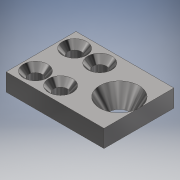
# Autodesk Inventor part: v2_bearing_insert_thick_round
Saved by Autodesk Inventor 2018 (Build 220112000, 112)
## iProperties
Created: 2017-04-27
Part Number: v2_bearing_insert_thick_round
Material: Stainless Steel, 440C
Document SubType Name: Modeling
Designer: richp
Density: 7.75 g/cm^3
Appearance: Semi-Polished
bearing_thickness: 0.125 in
Author: richp
Autodesk Inventor part; units mm, degrees
ref_plane "YZ Plane" through (0, 0, 0) normal (1, 0, 0) x (0, 1, 0)
sketch "Sketch1" plane through (0, 0, 0) normal (1, 0, 0) x (0, 1, 0)
  line L0 (-1.3067, 0) -> (7.8401, 0) construction
  line L1 (0, -10.9768) -> (0, 10.9768) construction
  line L2 (0, -1.7272) -> (0, -6.35)
  line L3 (0, -1.7272) -> (0, -1.7272)
  line L4 (0, -1.7272) -> (3.175, -3.5603)
  line L5 (3.175, -3.5603) -> (3.175, -6.35)
  line L6 (3.175, -6.35) -> (0, -6.35)
  circle A0 centre (3.3584, 0) radius 3.175 construction
  line L7 (2.5647, 7.8406) -> (4.1522, 7.8406) construction
  line L8 (4.1522, 7.8406) -> (4.1522, -7.8406) construction
  line L9 (4.1522, -7.8406) -> (2.5647, -7.8406) construction
  line L10 (2.5647, -7.8406) -> (2.5647, 7.8406) construction
  line L11 (2.5647, 7.8406) -> (4.1522, -7.8406) construction
  line L12 (4.1522, 7.8406) -> (2.5647, -7.8406) construction
  line L13 (0, 1.7272) -> (0, 6.35)
  line L14 (0, 1.7272) -> (0, 1.7272)
  line L15 (0, 1.7272) -> (3.175, 3.5603)
  line L16 (3.175, 3.5603) -> (3.175, 6.35)
  line L17 (3.175, 6.35) -> (0, 6.35)
  point P0 (0, 0)
  point P1 (2.3851, -3.0222)
  point P2 (2.3851, 3.0222)
  dimension "d12" = 60
  dimension "d13" = 0
  dimension "bearing_thickness" = 3.175
  dimension "d15" = 1.7272
  dimension "d17" = 6.35
  dimension "d18" = 1.5875
  dimension "d23" = 12.7
  dimension "d52" = 3.3584
  constraints: 32 end point, 5 symmetric about line, 4 perpendicular, 2 horizontal, 2 midpoint, 2 parallel, 2 point on circle, 2 point on line, 1 centre point, 1 coincident, 1 tangent
  measures "d12" angle of L1 L4
  measures "d13" distance of L2.start L3.end
  measures "bearing_thickness" distance of L5.end L2.end
  measures "d15" distance from line of point (0, 0) L3
  measures "d17" diameter of A0
  measures "d18" distance between parallel lines of L10 L8
  measures "d23" distance between parallel lines of L6 L17
  measures "d52" distance from line of L2 A0.centre
sketch "Sketch11" plane through (0, 0, 0) normal (1, 0, 0) x (0, 1, 0)
  line L0 (3.175, 6.35) -> (0, 6.35) projected
  line L1 (3.175, -6.35) -> (0, -6.35) projected
  line L2 (-1.3067, 0) -> (7.8401, 0) construction
  line L3 (0, -10.9768) -> (0, 10.9768) construction
  line L4 (3.175, 6.35) -> (3.175, 0.762)
  line L5 (3.175, 0.762) -> (0, 0.762)
  line L6 (0, 6.35) -> (0, 0.762)
  line L7 (3.175, -6.35) -> (0, -6.35)
  line L8 (0, 10.9768) -> (0, -10.9768) construction
  line L9 (3.175, -6.35) -> (3.175, -0.762)
  line L10 (3.175, -0.762) -> (0, -0.762)
  line L11 (0, -6.35) -> (0, -0.762)
  point P0 (0, 0)
  dimension "d54" = 5.588
  constraints: 16 end point, 4 symmetric about line, 2 perpendicular, 2 point on line, 1 vertical
  measures "d54" distance of L0.start L4.end
extrude "Extrusion4" add sketch "Sketch11" along normal blind 3.556 and the other way blind 14.224
sketch "Sketch17" plane through (3.556, 0, 0) normal (1, 0, 0) x (0, 0, -1)
  line L0 (-6.35, 3.175) -> (-0.762, 3.175) projected
  line L1 (-0.762, 3.175) -> (0.762, 3.175)
  line L2 (0.762, 3.175) -> (0.762, 0)
  line L3 (0.762, 0) -> (-0.762, 0)
  line L4 (-0.762, 0) -> (-0.762, 3.175)
  point P0 (0, 0)
  constraints: 8 end point, 2 parallel, 1 horizontal, 1 perpendicular
ref_plane "Work Plane3" through (0, 3.175, 6.35) normal (1, 0, 0) x (0, -1, 0)
extrude "Extrusion6" add sketch "Sketch17" against normal blind 17.78
sketch "Sketch14" plane through (-14.224, 3.175, -6.35) normal (0, 1, 0) x (1, 0, 0)
  line L0 (-3.556, -6.35) -> (21.336, -6.35) projected
  line L1 (0, -5.588) -> (0, 0) projected
  point P0 (14.224, -6.35)
  point P1 (2.54, -2.794)
  point P2 (7.112, -2.794)
  point P3 (2.54, -9.906)
  point P4 (7.112, -9.906)
  dimension "d65" = 7.112
  dimension "d66" = 11.684
  dimension "d67" = 3.556
  constraints: 2 symmetric about line, 1 horizontal alignment
  measures "d65" horizontal distance of point (7.112, -2.794) point (14.224, -6.35)
  measures "d66" horizontal distance of point (2.54, -2.794) point (14.224, -6.35)
  measures "d67" distance from line of L0 point (2.54, -2.794)
hole "Hole2" at (-11.684, 3.175, -3.556) at (-7.112, 3.175, -3.556) at (-11.684, 3.175, 3.556) at (-7.112, 3.175, 3.556) direction (0, -1, 0) diameter 2.4384 depth 6.6294 tip angle 118 countersink diameter 4.3688 countersink angle 82 clearance for "Flat Head Machine Screw (82)" size "#2" standard "Ansi Unified Screw Threads"
sketch "Sketch12" plane through (0, 3.175, 6.35) normal (1, 0, 0) x (0, -1, 0)
  line L0 (3.175, 4.6228) -> (0, 2.7897) projected
  line L1 (3.175, 8.0772) -> (0, 9.9103) projected
  line L2 (4.4817, 6.35) -> (-4.6651, 6.35) construction
  line L3 (3.175, 17.3268) -> (3.175, -4.6268) construction
  line L4 (3.175, 4.6228) -> (3.175, 7.0113)
  line L5 (3.175, 4.6228) -> (3.175, 4.6228)
  line L6 (3.175, 8.0772) -> (3.175, 8.0772)
  line L7 (3.175, 7.0113) -> (3.175, 8.0772)
  line L8 (0, 2.7897) -> (0, 9.9103)
  line L9 (0, 0) -> (0, 5.588) projected
  point P0 (3.175, 6.35)
  constraints: 10 end point, 4 collinear, 3 point on line
extrude "Extrusion5" [suppressed]
ref_plane "Work Plane4" through (0, 2.5647, -7.8406) normal (-1, 0, 0) x (0, 0, 1)
sketch "Sketch16" plane through (0, 2.5647, -7.8406) normal (-1, 0, 0) x (0, 0, 1)
  line L0 (6.1134, -2.5647) -> (4.2803, 0.6103) projected
  line L1 (9.5678, -2.5647) -> (11.4008, 0.6103) projected
  line L2 (11.4008, 0.6103) -> (4.2803, 0.6103) projected
  line L3 (7.1793, -2.5647) -> (6.1134, -2.5647) projected
  line L4 (9.5678, -2.5647) -> (7.1793, -2.5647) projected
  line L5 (9.5678, -2.5647) -> (9.5678, -2.5647)
  line L6 (6.1134, -2.5647) -> (6.1134, -2.5647)
  line L7 (7.8406, -3.8713) -> (7.8406, 5.2754) projected
  line L8 (7.8406, 0.6103) -> (7.8406, -2.5647)
  constraints: 6 end point, 1 collinear, 1 midpoint, 1 point on line
revolve "Revolution7" cut sketch "Sketch16" angle 360 about axis through (0, 3.175, 0) along (0, -1, 0) contours L2 L1 L4 L7
sketch "Sketch13" plane through (0, 3.175, 6.35) normal (1, 0, 0) x (0, -1, 0)
  circle A0 centre (-0.1834, 6.35) radius 3.175 projected
  line L0 (4.4817, 6.35) -> (-4.6651, 6.35) construction
  line L1 (-3.3584, 6.35) -> (2.9916, 6.35)
  point P0 (3.175, 6.35)
  constraints: 2 end point, 2 point on circle, 2 point on line
revolve "Revolution6" cut sketch "Sketch13" angle 360 about axis through (0, 6.5334, 0) along (0, -1, 0)
equation "\"d12\" = bearing_angle"
equation "\"d15\" = bearing_spacing"
equation "\"d65\" = hole1_setback"
equation "\"d66\" = hole2_setback"
equation "\"d67\" = hole_lateral"
equation "\"hole1_setback_qq\" = 7.112"
equation "\"hole_lateral_qq\" = 3.556"
equation "\"hole2_setback_qq\" = 11.684"
equation "\"bearing_angle_qq\" = 60deg"
equation "\"bearing_spacing_qq\" = 1.7272"
equation "\"bearing_angle\" = 60deg"
equation "\"bearing_spacing\" = 1.7272"
equation "\"hole1_setback\" = 7.112"
equation "\"hole2_setback\" = 11.684"
equation "\"hole_lateral\" = 3.556"
body "Solid2"
